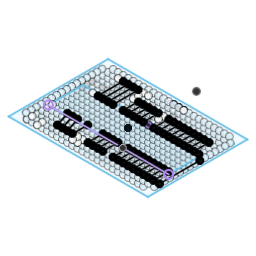
teensy_circuit_board v7 (Autodesk Fusion 360 design; units mm, degrees)
Autodesk Fusion 360 part; units mm, degrees
sketch "board" plane through (0, 0, 0) normal (0, 0, 1) x (1, 0, 0)
  circle A0 centre (-29.2, -21.5) radius 0.5
  line L0 (-35, 25) -> (35, 25)
  line L1 (35, 25) -> (35, -25)
  line L2 (35, -25) -> (-35, -25)
  line L3 (-35, -25) -> (-35, 25)
  circle A1 centre (-26.66, -21.5) radius 0.5
  circle A2 centre (-24.12, -21.5) radius 0.5
  circle A3 centre (-21.58, -21.5) radius 0.5
  circle A4 centre (-19.04, -21.5) radius 0.5
  circle A5 centre (-16.5, -21.5) radius 0.5
  circle A6 centre (-13.96, -21.5) radius 0.5
  circle A7 centre (-11.42, -21.5) radius 0.5
  circle A8 centre (-8.88, -21.5) radius 0.5
  circle A9 centre (-6.34, -21.5) radius 0.5
  circle A10 centre (-3.8, -21.5) radius 0.5
  circle A11 centre (-1.26, -21.5) radius 0.5
  circle A12 centre (1.28, -21.5) radius 0.5
  circle A13 centre (3.82, -21.5) radius 0.5
  circle A14 centre (6.36, -21.5) radius 0.5
  circle A15 centre (8.9, -21.5) radius 0.5
  circle A16 centre (11.44, -21.5) radius 0.5
  circle A17 centre (13.98, -21.5) radius 0.5
  circle A18 centre (16.52, -21.5) radius 0.5
  circle A19 centre (19.06, -21.5) radius 0.5
  circle A20 centre (21.6, -21.5) radius 0.5
  circle A21 centre (24.14, -21.5) radius 0.5
  circle A22 centre (26.68, -21.5) radius 0.5
  circle A23 centre (29.22, -21.5) radius 0.5
  circle A24 centre (-29.2, -18.96) radius 0.5
  circle A25 centre (-26.66, -18.96) radius 0.5
  circle A26 centre (-24.12, -18.96) radius 0.5
  circle A27 centre (-21.58, -18.96) radius 0.5
  circle A28 centre (-19.04, -18.96) radius 0.5
  circle A29 centre (-16.5, -18.96) radius 0.5
  circle A30 centre (-13.96, -18.96) radius 0.5
  circle A31 centre (-11.42, -18.96) radius 0.5
  circle A32 centre (-8.88, -18.96) radius 0.5
  circle A33 centre (-6.34, -18.96) radius 0.5
  circle A34 centre (-3.8, -18.96) radius 0.5
  circle A35 centre (-1.26, -18.96) radius 0.5
  circle A36 centre (1.28, -18.96) radius 0.5
  circle A37 centre (3.82, -18.96) radius 0.5
  circle A38 centre (6.36, -18.96) radius 0.5
  circle A39 centre (8.9, -18.96) radius 0.5
  circle A40 centre (11.44, -18.96) radius 0.5
  circle A41 centre (13.98, -18.96) radius 0.5
  circle A42 centre (16.52, -18.96) radius 0.5
  circle A43 centre (19.06, -18.96) radius 0.5
  circle A44 centre (21.6, -18.96) radius 0.5
  circle A45 centre (24.14, -18.96) radius 0.5
  circle A46 centre (26.68, -18.96) radius 0.5
  circle A47 centre (29.22, -18.96) radius 0.5
  circle A48 centre (-29.2, -16.42) radius 0.5
  circle A49 centre (-26.66, -16.42) radius 0.5
  circle A50 centre (-24.12, -16.42) radius 0.5
  circle A51 centre (-21.58, -16.42) radius 0.5
  circle A52 centre (-19.04, -16.42) radius 0.5
  circle A53 centre (-16.5, -16.42) radius 0.5
  circle A54 centre (-13.96, -16.42) radius 0.5
  circle A55 centre (-11.42, -16.42) radius 0.5
  circle A56 centre (-8.88, -16.42) radius 0.5
  circle A57 centre (-6.34, -16.42) radius 0.5
  circle A58 centre (-3.8, -16.42) radius 0.5
  circle A59 centre (-1.26, -16.42) radius 0.5
  circle A60 centre (1.28, -16.42) radius 0.5
  circle A61 centre (3.82, -16.42) radius 0.5
  circle A62 centre (6.36, -16.42) radius 0.5
  circle A63 centre (8.9, -16.42) radius 0.5
  circle A64 centre (11.44, -16.42) radius 0.5
  circle A65 centre (13.98, -16.42) radius 0.5
  circle A66 centre (16.52, -16.42) radius 0.5
  circle A67 centre (19.06, -16.42) radius 0.5
  circle A68 centre (21.6, -16.42) radius 0.5
  circle A69 centre (24.14, -16.42) radius 0.5
  circle A70 centre (26.68, -16.42) radius 0.5
  circle A71 centre (29.22, -16.42) radius 0.5
  circle A72 centre (-29.2, -13.88) radius 0.5
  circle A73 centre (-26.66, -13.88) radius 0.5
  circle A74 centre (-24.12, -13.88) radius 0.5
  circle A75 centre (-21.58, -13.88) radius 0.5
  circle A76 centre (-19.04, -13.88) radius 0.5
  circle A77 centre (-16.5, -13.88) radius 0.5
  circle A78 centre (-13.96, -13.88) radius 0.5
  circle A79 centre (-11.42, -13.88) radius 0.5
  circle A80 centre (-8.88, -13.88) radius 0.5
  circle A81 centre (-6.34, -13.88) radius 0.5
  circle A82 centre (-3.8, -13.88) radius 0.5
  circle A83 centre (-1.26, -13.88) radius 0.5
  circle A84 centre (1.28, -13.88) radius 0.5
  circle A85 centre (3.82, -13.88) radius 0.5
  circle A86 centre (6.36, -13.88) radius 0.5
  circle A87 centre (8.9, -13.88) radius 0.5
  circle A88 centre (11.44, -13.88) radius 0.5
  circle A89 centre (13.98, -13.88) radius 0.5
  circle A90 centre (16.52, -13.88) radius 0.5
  circle A91 centre (19.06, -13.88) radius 0.5
  circle A92 centre (21.6, -13.88) radius 0.5
  circle A93 centre (24.14, -13.88) radius 0.5
  circle A94 centre (26.68, -13.88) radius 0.5
  circle A95 centre (29.22, -13.88) radius 0.5
  circle A96 centre (-29.2, -11.34) radius 0.5
  circle A97 centre (-26.66, -11.34) radius 0.5
  circle A98 centre (-24.12, -11.34) radius 0.5
  circle A99 centre (-21.58, -11.34) radius 0.5
  circle A100 centre (-19.04, -11.34) radius 0.5
  circle A101 centre (-16.5, -11.34) radius 0.5
  circle A102 centre (-13.96, -11.34) radius 0.5
  circle A103 centre (-11.42, -11.34) radius 0.5
  circle A104 centre (-8.88, -11.34) radius 0.5
  circle A105 centre (-6.34, -11.34) radius 0.5
  circle A106 centre (-3.8, -11.34) radius 0.5
  circle A107 centre (-1.26, -11.34) radius 0.5
  circle A108 centre (1.28, -11.34) radius 0.5
  circle A109 centre (3.82, -11.34) radius 0.5
  circle A110 centre (6.36, -11.34) radius 0.5
  circle A111 centre (8.9, -11.34) radius 0.5
  circle A112 centre (11.44, -11.34) radius 0.5
  circle A113 centre (13.98, -11.34) radius 0.5
  circle A114 centre (16.52, -11.34) radius 0.5
  circle A115 centre (19.06, -11.34) radius 0.5
  circle A116 centre (21.6, -11.34) radius 0.5
  circle A117 centre (24.14, -11.34) radius 0.5
  circle A118 centre (26.68, -11.34) radius 0.5
  circle A119 centre (29.22, -11.34) radius 0.5
  circle A120 centre (-29.2, -8.8) radius 0.5
  circle A121 centre (-26.66, -8.8) radius 0.5
  circle A122 centre (-24.12, -8.8) radius 0.5
  circle A123 centre (-21.58, -8.8) radius 0.5
  circle A124 centre (-19.04, -8.8) radius 0.5
  circle A125 centre (-16.5, -8.8) radius 0.5
  circle A126 centre (-13.96, -8.8) radius 0.5
  circle A127 centre (-11.42, -8.8) radius 0.5
  circle A128 centre (-8.88, -8.8) radius 0.5
  circle A129 centre (-6.34, -8.8) radius 0.5
  circle A130 centre (-3.8, -8.8) radius 0.5
  circle A131 centre (-1.26, -8.8) radius 0.5
  circle A132 centre (1.28, -8.8) radius 0.5
  circle A133 centre (3.82, -8.8) radius 0.5
  circle A134 centre (6.36, -8.8) radius 0.5
  circle A135 centre (8.9, -8.8) radius 0.5
  circle A136 centre (11.44, -8.8) radius 0.5
  circle A137 centre (13.98, -8.8) radius 0.5
  circle A138 centre (16.52, -8.8) radius 0.5
  circle A139 centre (19.06, -8.8) radius 0.5
  circle A140 centre (21.6, -8.8) radius 0.5
  circle A141 centre (24.14, -8.8) radius 0.5
  circle A142 centre (26.68, -8.8) radius 0.5
  circle A143 centre (29.22, -8.8) radius 0.5
  circle A144 centre (-29.2, -6.26) radius 0.5
  circle A145 centre (-26.66, -6.26) radius 0.5
  circle A146 centre (-24.12, -6.26) radius 0.5
  circle A147 centre (-21.58, -6.26) radius 0.5
  circle A148 centre (-19.04, -6.26) radius 0.5
  circle A149 centre (-16.5, -6.26) radius 0.5
  circle A150 centre (-13.96, -6.26) radius 0.5
  circle A151 centre (-11.42, -6.26) radius 0.5
  circle A152 centre (-8.88, -6.26) radius 0.5
  circle A153 centre (-6.34, -6.26) radius 0.5
  circle A154 centre (-3.8, -6.26) radius 0.5
  circle A155 centre (-1.26, -6.26) radius 0.5
  circle A156 centre (1.28, -6.26) radius 0.5
  circle A157 centre (3.82, -6.26) radius 0.5
  circle A158 centre (6.36, -6.26) radius 0.5
  circle A159 centre (8.9, -6.26) radius 0.5
  circle A160 centre (11.44, -6.26) radius 0.5
  circle A161 centre (13.98, -6.26) radius 0.5
  circle A162 centre (16.52, -6.26) radius 0.5
  circle A163 centre (19.06, -6.26) radius 0.5
  circle A164 centre (21.6, -6.26) radius 0.5
  circle A165 centre (24.14, -6.26) radius 0.5
  circle A166 centre (26.68, -6.26) radius 0.5
  circle A167 centre (29.22, -6.26) radius 0.5
  circle A168 centre (-29.2, -3.72) radius 0.5
  circle A169 centre (-26.66, -3.72) radius 0.5
  circle A170 centre (-24.12, -3.72) radius 0.5
  circle A171 centre (-21.58, -3.72) radius 0.5
  circle A172 centre (-19.04, -3.72) radius 0.5
  circle A173 centre (-16.5, -3.72) radius 0.5
  circle A174 centre (-13.96, -3.72) radius 0.5
  circle A175 centre (-11.42, -3.72) radius 0.5
  circle A176 centre (-8.88, -3.72) radius 0.5
  circle A177 centre (-6.34, -3.72) radius 0.5
  circle A178 centre (-3.8, -3.72) radius 0.5
  circle A179 centre (-1.26, -3.72) radius 0.5
  circle A180 centre (1.28, -3.72) radius 0.5
  circle A181 centre (3.82, -3.72) radius 0.5
  circle A182 centre (6.36, -3.72) radius 0.5
  circle A183 centre (8.9, -3.72) radius 0.5
  circle A184 centre (11.44, -3.72) radius 0.5
  circle A185 centre (13.98, -3.72) radius 0.5
  circle A186 centre (16.52, -3.72) radius 0.5
  circle A187 centre (19.06, -3.72) radius 0.5
  circle A188 centre (21.6, -3.72) radius 0.5
  circle A189 centre (24.14, -3.72) radius 0.5
  circle A190 centre (26.68, -3.72) radius 0.5
  circle A191 centre (29.22, -3.72) radius 0.5
  circle A192 centre (-29.2, -1.18) radius 0.5
  circle A193 centre (-26.66, -1.18) radius 0.5
  circle A194 centre (-24.12, -1.18) radius 0.5
  circle A195 centre (-21.58, -1.18) radius 0.5
  circle A196 centre (-19.04, -1.18) radius 0.5
  circle A197 centre (-16.5, -1.18) radius 0.5
  circle A198 centre (-13.96, -1.18) radius 0.5
  circle A199 centre (-11.42, -1.18) radius 0.5
  circle A200 centre (-8.88, -1.18) radius 0.5
  circle A201 centre (-6.34, -1.18) radius 0.5
  circle A202 centre (-3.8, -1.18) radius 0.5
  circle A203 centre (-1.26, -1.18) radius 0.5
  circle A204 centre (1.28, -1.18) radius 0.5
  circle A205 centre (3.82, -1.18) radius 0.5
  circle A206 centre (6.36, -1.18) radius 0.5
  circle A207 centre (8.9, -1.18) radius 0.5
  circle A208 centre (11.44, -1.18) radius 0.5
  circle A209 centre (13.98, -1.18) radius 0.5
  circle A210 centre (16.52, -1.18) radius 0.5
  circle A211 centre (19.06, -1.18) radius 0.5
  circle A212 centre (21.6, -1.18) radius 0.5
  circle A213 centre (24.14, -1.18) radius 0.5
  circle A214 centre (26.68, -1.18) radius 0.5
  circle A215 centre (29.22, -1.18) radius 0.5
  circle A216 centre (-29.2, 1.36) radius 0.5
  circle A217 centre (-26.66, 1.36) radius 0.5
  circle A218 centre (-24.12, 1.36) radius 0.5
  circle A219 centre (-21.58, 1.36) radius 0.5
  circle A220 centre (-19.04, 1.36) radius 0.5
  circle A221 centre (-16.5, 1.36) radius 0.5
  circle A222 centre (-13.96, 1.36) radius 0.5
  circle A223 centre (-11.42, 1.36) radius 0.5
  circle A224 centre (-8.88, 1.36) radius 0.5
  circle A225 centre (-6.34, 1.36) radius 0.5
  circle A226 centre (-3.8, 1.36) radius 0.5
  circle A227 centre (-1.26, 1.36) radius 0.5
  circle A228 centre (1.28, 1.36) radius 0.5
  circle A229 centre (3.82, 1.36) radius 0.5
  circle A230 centre (6.36, 1.36) radius 0.5
  circle A231 centre (8.9, 1.36) radius 0.5
  circle A232 centre (11.44, 1.36) radius 0.5
  circle A233 centre (13.98, 1.36) radius 0.5
  circle A234 centre (16.52, 1.36) radius 0.5
  circle A235 centre (19.06, 1.36) radius 0.5
  circle A236 centre (21.6, 1.36) radius 0.5
  circle A237 centre (24.14, 1.36) radius 0.5
  circle A238 centre (26.68, 1.36) radius 0.5
  circle A239 centre (29.22, 1.36) radius 0.5
  circle A240 centre (-29.2, 3.9) radius 0.5
  circle A241 centre (-26.66, 3.9) radius 0.5
  circle A242 centre (-24.12, 3.9) radius 0.5
  circle A243 centre (-21.58, 3.9) radius 0.5
  circle A244 centre (-19.04, 3.9) radius 0.5
  circle A245 centre (-16.5, 3.9) radius 0.5
  circle A246 centre (-13.96, 3.9) radius 0.5
  circle A247 centre (-11.42, 3.9) radius 0.5
  circle A248 centre (-8.88, 3.9) radius 0.5
  circle A249 centre (-6.34, 3.9) radius 0.5
  circle A250 centre (-3.8, 3.9) radius 0.5
  circle A251 centre (-1.26, 3.9) radius 0.5
  circle A252 centre (1.28, 3.9) radius 0.5
  circle A253 centre (3.82, 3.9) radius 0.5
  circle A254 centre (6.36, 3.9) radius 0.5
  circle A255 centre (8.9, 3.9) radius 0.5
  circle A256 centre (11.44, 3.9) radius 0.5
  circle A257 centre (13.98, 3.9) radius 0.5
  circle A258 centre (16.52, 3.9) radius 0.5
  circle A259 centre (19.06, 3.9) radius 0.5
  circle A260 centre (21.6, 3.9) radius 0.5
  circle A261 centre (24.14, 3.9) radius 0.5
  circle A262 centre (26.68, 3.9) radius 0.5
  circle A263 centre (29.22, 3.9) radius 0.5
  circle A264 centre (-29.2, 6.44) radius 0.5
  circle A265 centre (-26.66, 6.44) radius 0.5
  circle A266 centre (-24.12, 6.44) radius 0.5
  circle A267 centre (-21.58, 6.44) radius 0.5
  circle A268 centre (-19.04, 6.44) radius 0.5
  circle A269 centre (-16.5, 6.44) radius 0.5
  circle A270 centre (-13.96, 6.44) radius 0.5
  circle A271 centre (-11.42, 6.44) radius 0.5
  circle A272 centre (-8.88, 6.44) radius 0.5
  circle A273 centre (-6.34, 6.44) radius 0.5
  circle A274 centre (-3.8, 6.44) radius 0.5
  circle A275 centre (-1.26, 6.44) radius 0.5
  circle A276 centre (1.28, 6.44) radius 0.5
  circle A277 centre (3.82, 6.44) radius 0.5
  circle A278 centre (6.36, 6.44) radius 0.5
  circle A279 centre (8.9, 6.44) radius 0.5
  circle A280 centre (11.44, 6.44) radius 0.5
  circle A281 centre (13.98, 6.44) radius 0.5
  circle A282 centre (16.52, 6.44) radius 0.5
  circle A283 centre (19.06, 6.44) radius 0.5
  circle A284 centre (21.6, 6.44) radius 0.5
  circle A285 centre (24.14, 6.44) radius 0.5
  circle A286 centre (26.68, 6.44) radius 0.5
  circle A287 centre (29.22, 6.44) radius 0.5
  circle A288 centre (-29.2, 8.98) radius 0.5
  circle A289 centre (-26.66, 8.98) radius 0.5
  circle A290 centre (-24.12, 8.98) radius 0.5
  circle A291 centre (-21.58, 8.98) radius 0.5
  circle A292 centre (-19.04, 8.98) radius 0.5
  circle A293 centre (-16.5, 8.98) radius 0.5
  circle A294 centre (-13.96, 8.98) radius 0.5
  circle A295 centre (-11.42, 8.98) radius 0.5
  circle A296 centre (-8.88, 8.98) radius 0.5
  circle A297 centre (-6.34, 8.98) radius 0.5
  circle A298 centre (-3.8, 8.98) radius 0.5
  circle A299 centre (-1.26, 8.98) radius 0.5
  circle A300 centre (1.28, 8.98) radius 0.5
  circle A301 centre (3.82, 8.98) radius 0.5
  circle A302 centre (6.36, 8.98) radius 0.5
  circle A303 centre (8.9, 8.98) radius 0.5
  circle A304 centre (11.44, 8.98) radius 0.5
  circle A305 centre (13.98, 8.98) radius 0.5
  circle A306 centre (16.52, 8.98) radius 0.5
  circle A307 centre (19.06, 8.98) radius 0.5
  circle A308 centre (21.6, 8.98) radius 0.5
  circle A309 centre (24.14, 8.98) radius 0.5
  circle A310 centre (26.68, 8.98) radius 0.5
  circle A311 centre (29.22, 8.98) radius 0.5
  circle A312 centre (-29.2, 11.52) radius 0.5
  circle A313 centre (-26.66, 11.52) radius 0.5
  circle A314 centre (-24.12, 11.52) radius 0.5
  circle A315 centre (-21.58, 11.52) radius 0.5
  circle A316 centre (-19.04, 11.52) radius 0.5
  circle A317 centre (-16.5, 11.52) radius 0.5
  circle A318 centre (-13.96, 11.52) radius 0.5
  circle A319 centre (-11.42, 11.52) radius 0.5
  circle A320 centre (-8.88, 11.52) radius 0.5
  circle A321 centre (-6.34, 11.52) radius 0.5
  circle A322 centre (-3.8, 11.52) radius 0.5
  circle A323 centre (-1.26, 11.52) radius 0.5
  circle A324 centre (1.28, 11.52) radius 0.5
  circle A325 centre (3.82, 11.52) radius 0.5
  circle A326 centre (6.36, 11.52) radius 0.5
  circle A327 centre (8.9, 11.52) radius 0.5
  circle A328 centre (11.44, 11.52) radius 0.5
  circle A329 centre (13.98, 11.52) radius 0.5
  circle A330 centre (16.52, 11.52) radius 0.5
  circle A331 centre (19.06, 11.52) radius 0.5
  circle A332 centre (21.6, 11.52) radius 0.5
  circle A333 centre (24.14, 11.52) radius 0.5
  circle A334 centre (26.68, 11.52) radius 0.5
  circle A335 centre (29.22, 11.52) radius 0.5
  circle A336 centre (-29.2, 14.06) radius 0.5
  circle A337 centre (-26.66, 14.06) radius 0.5
  circle A338 centre (-24.12, 14.06) radius 0.5
  circle A339 centre (-21.58, 14.06) radius 0.5
  circle A340 centre (-19.04, 14.06) radius 0.5
  circle A341 centre (-16.5, 14.06) radius 0.5
  circle A342 centre (-13.96, 14.06) radius 0.5
  circle A343 centre (-11.42, 14.06) radius 0.5
  circle A344 centre (-8.88, 14.06) radius 0.5
  circle A345 centre (-6.34, 14.06) radius 0.5
  circle A346 centre (-3.8, 14.06) radius 0.5
  circle A347 centre (-1.26, 14.06) radius 0.5
  circle A348 centre (1.28, 14.06) radius 0.5
  circle A349 centre (3.82, 14.06) radius 0.5
  circle A350 centre (6.36, 14.06) radius 0.5
  circle A351 centre (8.9, 14.06) radius 0.5
  circle A352 centre (11.44, 14.06) radius 0.5
  circle A353 centre (13.98, 14.06) radius 0.5
  circle A354 centre (16.52, 14.06) radius 0.5
  circle A355 centre (19.06, 14.06) radius 0.5
  circle A356 centre (21.6, 14.06) radius 0.5
  circle A357 centre (24.14, 14.06) radius 0.5
  circle A358 centre (26.68, 14.06) radius 0.5
  circle A359 centre (29.22, 14.06) radius 0.5
  circle A360 centre (-29.2, 16.6) radius 0.5
  circle A361 centre (-26.66, 16.6) radius 0.5
  circle A362 centre (-24.12, 16.6) radius 0.5
  circle A363 centre (-21.58, 16.6) radius 0.5
  circle A364 centre (-19.04, 16.6) radius 0.5
  circle A365 centre (-16.5, 16.6) radius 0.5
  circle A366 centre (-13.96, 16.6) radius 0.5
  circle A367 centre (-11.42, 16.6) radius 0.5
  circle A368 centre (-8.88, 16.6) radius 0.5
  circle A369 centre (-6.34, 16.6) radius 0.5
  circle A370 centre (-3.8, 16.6) radius 0.5
  circle A371 centre (-1.26, 16.6) radius 0.5
  circle A372 centre (1.28, 16.6) radius 0.5
  circle A373 centre (3.82, 16.6) radius 0.5
  circle A374 centre (6.36, 16.6) radius 0.5
  circle A375 centre (8.9, 16.6) radius 0.5
  circle A376 centre (11.44, 16.6) radius 0.5
  circle A377 centre (13.98, 16.6) radius 0.5
  circle A378 centre (16.52, 16.6) radius 0.5
  circle A379 centre (19.06, 16.6) radius 0.5
  circle A380 centre (21.6, 16.6) radius 0.5
  circle A381 centre (24.14, 16.6) radius 0.5
  circle A382 centre (26.68, 16.6) radius 0.5
  circle A383 centre (29.22, 16.6) radius 0.5
  circle A384 centre (-29.2, 19.14) radius 0.5
  circle A385 centre (-26.66, 19.14) radius 0.5
  circle A386 centre (-24.12, 19.14) radius 0.5
  circle A387 centre (-21.58, 19.14) radius 0.5
  circle A388 centre (-19.04, 19.14) radius 0.5
  circle A389 centre (-16.5, 19.14) radius 0.5
  circle A390 centre (-13.96, 19.14) radius 0.5
  circle A391 centre (-11.42, 19.14) radius 0.5
  circle A392 centre (-8.88, 19.14) radius 0.5
  circle A393 centre (-6.34, 19.14) radius 0.5
  circle A394 centre (-3.8, 19.14) radius 0.5
  circle A395 centre (-1.26, 19.14) radius 0.5
  circle A396 centre (1.28, 19.14) radius 0.5
  circle A397 centre (3.82, 19.14) radius 0.5
  circle A398 centre (6.36, 19.14) radius 0.5
  circle A399 centre (8.9, 19.14) radius 0.5
  circle A400 centre (11.44, 19.14) radius 0.5
  circle A401 centre (13.98, 19.14) radius 0.5
  circle A402 centre (16.52, 19.14) radius 0.5
  circle A403 centre (19.06, 19.14) radius 0.5
  circle A404 centre (21.6, 19.14) radius 0.5
  circle A405 centre (24.14, 19.14) radius 0.5
  circle A406 centre (26.68, 19.14) radius 0.5
  circle A407 centre (29.22, 19.14) radius 0.5
  circle A408 centre (-29.2, 21.68) radius 0.5
  circle A409 centre (-26.66, 21.68) radius 0.5
  circle A410 centre (-24.12, 21.68) radius 0.5
  circle A411 centre (-21.58, 21.68) radius 0.5
  circle A412 centre (-19.04, 21.68) radius 0.5
  circle A413 centre (-16.5, 21.68) radius 0.5
  circle A414 centre (-13.96, 21.68) radius 0.5
  circle A415 centre (-11.42, 21.68) radius 0.5
  circle A416 centre (-8.88, 21.68) radius 0.5
  circle A417 centre (-6.34, 21.68) radius 0.5
  circle A418 centre (-3.8, 21.68) radius 0.5
  circle A419 centre (-1.26, 21.68) radius 0.5
  circle A420 centre (1.28, 21.68) radius 0.5
  circle A421 centre (3.82, 21.68) radius 0.5
  circle A422 centre (6.36, 21.68) radius 0.5
  circle A423 centre (8.9, 21.68) radius 0.5
  circle A424 centre (11.44, 21.68) radius 0.5
  circle A425 centre (13.98, 21.68) radius 0.5
  circle A426 centre (16.52, 21.68) radius 0.5
  circle A427 centre (19.06, 21.68) radius 0.5
  circle A428 centre (21.6, 21.68) radius 0.5
  circle A429 centre (24.14, 21.68) radius 0.5
  circle A430 centre (26.68, 21.68) radius 0.5
  circle A431 centre (29.22, 21.68) radius 0.5
  line L4 (-33.3, 18.5) -> (-33.3, 19.8)
  line L5 (-33.3, 19.8) -> (-32.2, 19.8)
  line L6 (-33.3, 18.5) -> (-32.2, 18.5)
  arc A432 (-32.2, 18.5) -> (-32.2, 19.8) centre (-32.2, 19.15) ccw
  arc A433 (-32.2, 15.96) -> (-32.2, 17.26) centre (-32.2, 16.61) ccw
  line L7 (-33.3, 15.96) -> (-32.2, 15.96)
  line L8 (-33.3, 15.96) -> (-33.3, 17.26)
  line L9 (-33.3, 17.26) -> (-32.2, 17.26)
  arc A434 (-32.2, 13.42) -> (-32.2, 14.72) centre (-32.2, 14.07) ccw
  line L10 (-33.3, 13.42) -> (-32.2, 13.42)
  line L11 (-33.3, 13.42) -> (-33.3, 14.72)
  line L12 (-33.3, 14.72) -> (-32.2, 14.72)
  arc A435 (-32.2, 10.88) -> (-32.2, 12.18) centre (-32.2, 11.53) ccw
  line L13 (-33.3, 10.88) -> (-32.2, 10.88)
  line L14 (-33.3, 10.88) -> (-33.3, 12.18)
  line L15 (-33.3, 12.18) -> (-32.2, 12.18)
  arc A436 (-32.2, 8.34) -> (-32.2, 9.64) centre (-32.2, 8.99) ccw
  line L16 (-33.3, 8.34) -> (-32.2, 8.34)
  line L17 (-33.3, 8.34) -> (-33.3, 9.64)
  line L18 (-33.3, 9.64) -> (-32.2, 9.64)
  arc A437 (-32.2, 5.8) -> (-32.2, 7.1) centre (-32.2, 6.45) ccw
  line L19 (-33.3, 5.8) -> (-32.2, 5.8)
  line L20 (-33.3, 5.8) -> (-33.3, 7.1)
  line L21 (-33.3, 7.1) -> (-32.2, 7.1)
  arc A438 (-32.2, 3.26) -> (-32.2, 4.56) centre (-32.2, 3.91) ccw
  line L22 (-33.3, 3.26) -> (-32.2, 3.26)
  line L23 (-33.3, 3.26) -> (-33.3, 4.56)
  line L24 (-33.3, 4.56) -> (-32.2, 4.56)
  arc A439 (-32.2, 0.72) -> (-32.2, 2.02) centre (-32.2, 1.37) ccw
  line L25 (-33.3, 0.72) -> (-32.2, 0.72)
  line L26 (-33.3, 0.72) -> (-33.3, 2.02)
  line L27 (-33.3, 2.02) -> (-32.2, 2.02)
  arc A440 (-32.2, -1.82) -> (-32.2, -0.52) centre (-32.2, -1.17) ccw
  line L28 (-33.3, -1.82) -> (-32.2, -1.82)
  line L29 (-33.3, -1.82) -> (-33.3, -0.52)
  line L30 (-33.3, -0.52) -> (-32.2, -0.52)
  arc A441 (-32.2, -4.36) -> (-32.2, -3.06) centre (-32.2, -3.71) ccw
  line L31 (-33.3, -4.36) -> (-32.2, -4.36)
  line L32 (-33.3, -4.36) -> (-33.3, -3.06)
  line L33 (-33.3, -3.06) -> (-32.2, -3.06)
  arc A442 (-32.2, -6.9) -> (-32.2, -5.6) centre (-32.2, -6.25) ccw
  line L34 (-33.3, -6.9) -> (-32.2, -6.9)
  line L35 (-33.3, -6.9) -> (-33.3, -5.6)
  line L36 (-33.3, -5.6) -> (-32.2, -5.6)
  arc A443 (-32.2, -9.44) -> (-32.2, -8.14) centre (-32.2, -8.79) ccw
  line L37 (-33.3, -9.44) -> (-32.2, -9.44)
  line L38 (-33.3, -9.44) -> (-33.3, -8.14)
  line L39 (-33.3, -8.14) -> (-32.2, -8.14)
  arc A444 (-32.2, -11.98) -> (-32.2, -10.68) centre (-32.2, -11.33) ccw
  line L40 (-33.3, -11.98) -> (-32.2, -11.98)
  line L41 (-33.3, -11.98) -> (-33.3, -10.68)
  line L42 (-33.3, -10.68) -> (-32.2, -10.68)
  arc A445 (-32.2, -14.52) -> (-32.2, -13.22) centre (-32.2, -13.87) ccw
  line L43 (-33.3, -14.52) -> (-32.2, -14.52)
  line L44 (-33.3, -14.52) -> (-33.3, -13.22)
  line L45 (-33.3, -13.22) -> (-32.2, -13.22)
  arc A446 (-32.2, -17.06) -> (-32.2, -15.76) centre (-32.2, -16.41) ccw
  line L46 (-33.3, -17.06) -> (-32.2, -17.06)
  line L47 (-33.3, -17.06) -> (-33.3, -15.76)
  line L48 (-33.3, -15.76) -> (-32.2, -15.76)
  arc A447 (-32.2, -19.6) -> (-32.2, -18.3) centre (-32.2, -18.95) ccw
  line L49 (-33.3, -19.6) -> (-32.2, -19.6)
  line L50 (-33.3, -19.6) -> (-33.3, -18.3)
  line L51 (-33.3, -18.3) -> (-32.2, -18.3)
  line L52 (33.3, -5.6) -> (32.2, -5.6)
  line L53 (33.3, 15.96) -> (32.2, 15.96)
  line L54 (33.3, 13.42) -> (32.2, 13.42)
  arc A448 (32.2, -13.22) -> (32.2, -14.52) centre (32.2, -13.87) ccw
  arc A449 (32.2, 19.8) -> (32.2, 18.5) centre (32.2, 19.15) ccw
  line L55 (33.3, -19.6) -> (33.3, -18.3)
  line L56 (33.3, 19.8) -> (32.2, 19.8)
  line L57 (33.3, 18.5) -> (32.2, 18.5)
  line L58 (33.3, 18.5) -> (33.3, 19.8)
  line L59 (33.3, 13.42) -> (33.3, 14.72)
  line L60 (33.3, -11.98) -> (33.3, -10.68)
  line L61 (33.3, -17.06) -> (32.2, -17.06)
  arc A450 (32.2, -10.68) -> (32.2, -11.98) centre (32.2, -11.33) ccw
  line L62 (33.3, 0.72) -> (33.3, 2.02)
  line L63 (33.3, 8.34) -> (33.3, 9.64)
  arc A451 (32.2, -8.14) -> (32.2, -9.44) centre (32.2, -8.79) ccw
  line L64 (33.3, -9.44) -> (33.3, -8.14)
  line L65 (33.3, -8.14) -> (32.2, -8.14)
  line L66 (33.3, 10.88) -> (32.2, 10.88)
  line L67 (33.3, -1.82) -> (32.2, -1.82)
  arc A452 (32.2, 2.02) -> (32.2, 0.72) centre (32.2, 1.37) ccw
  line L68 (33.3, -6.9) -> (32.2, -6.9)
  line L69 (33.3, -4.36) -> (32.2, -4.36)
  line L70 (33.3, 3.26) -> (33.3, 4.56)
  arc A453 (32.2, -5.6) -> (32.2, -6.9) centre (32.2, -6.25) ccw
  line L71 (33.3, 5.8) -> (33.3, 7.1)
  line L72 (33.3, -4.36) -> (33.3, -3.06)
  line L73 (33.3, 9.64) -> (32.2, 9.64)
  line L74 (33.3, 0.72) -> (32.2, 0.72)
  line L75 (33.3, 3.26) -> (32.2, 3.26)
  arc A454 (32.2, 9.64) -> (32.2, 8.34) centre (32.2, 8.99) ccw
  line L76 (33.3, -1.82) -> (33.3, -0.52)
  arc A455 (32.2, -0.52) -> (32.2, -1.82) centre (32.2, -1.17) ccw
  arc A456 (32.2, 4.56) -> (32.2, 3.26) centre (32.2, 3.91) ccw
  line L77 (33.3, 5.8) -> (32.2, 5.8)
  line L78 (33.3, -3.06) -> (32.2, -3.06)
  line L79 (33.3, -9.44) -> (32.2, -9.44)
  line L80 (33.3, 7.1) -> (32.2, 7.1)
  line L81 (33.3, 2.02) -> (32.2, 2.02)
  line L82 (33.3, -6.9) -> (33.3, -5.6)
  line L83 (33.3, -10.68) -> (32.2, -10.68)
  arc A457 (32.2, -3.06) -> (32.2, -4.36) centre (32.2, -3.71) ccw
  line L84 (33.3, 8.34) -> (32.2, 8.34)
  arc A458 (32.2, 7.1) -> (32.2, 5.8) centre (32.2, 6.45) ccw
  line L85 (33.3, -0.52) -> (32.2, -0.52)
  line L86 (33.3, 4.56) -> (32.2, 4.56)
  arc A459 (32.2, -15.76) -> (32.2, -17.06) centre (32.2, -16.41) ccw
  line L87 (33.3, -17.06) -> (33.3, -15.76)
  line L88 (33.3, -11.98) -> (32.2, -11.98)
  line L89 (33.3, 15.96) -> (33.3, 17.26)
  line L90 (33.3, -14.52) -> (33.3, -13.22)
  line L91 (33.3, -19.6) -> (32.2, -19.6)
  line L92 (33.3, 10.88) -> (33.3, 12.18)
  line L93 (33.3, 17.26) -> (32.2, 17.26)
  arc A460 (32.2, 17.26) -> (32.2, 15.96) centre (32.2, 16.61) ccw
  line L94 (33.3, -14.52) -> (32.2, -14.52)
  line L95 (33.3, -15.76) -> (32.2, -15.76)
  arc A461 (32.2, -18.3) -> (32.2, -19.6) centre (32.2, -18.95) ccw
  line L96 (33.3, 12.18) -> (32.2, 12.18)
  line L97 (33.3, -13.22) -> (32.2, -13.22)
  line L98 (33.3, 14.72) -> (32.2, 14.72)
  arc A462 (32.2, 12.18) -> (32.2, 10.88) centre (32.2, 11.53) ccw
  arc A463 (32.2, 14.72) -> (32.2, 13.42) centre (32.2, 14.07) ccw
  line L99 (33.3, -18.3) -> (32.2, -18.3)
  dimension "d1" = 70
  dimension "d2" = 50
  constraint horizontal L0
  constraint perpendicular L0 L1
  constraint parallel L0 L2
  constraint parallel L1 L3
  measures "d1" distance of L1.end L2.end
  measures "d2" distance of L0.end L1.end
sketch "teensy" plane through (0, 0, 0) normal (0, 0, 1) x (1, 0, 0)
  line L0 (-30, 7.5) -> (30.389, 7.5)
  line L1 (30.389, 7.5) -> (30.389, -10)
  line L2 (30.389, -10) -> (-30, -10)
  line L3 (-30, -10) -> (-30, 7.5)
  dimension "d11" = 17.5
  constraint horizontal L0
  constraint vertical L1
  constraint horizontal L2
  constraint vertical L3
  measures "d11" distance of L0.start L2.end
extrude "Extrude1" add sketch "teensy" against normal blind 1
sketch "connectors" plane through (0, 0, 0) normal (0, 0, 1) x (1, 0, 0)
  line L0 (-30.5809, -18.0287) -> (-23.3364, -18.0287)
  line L1 (-23.3364, -18.0287) -> (-23.3364, -19.8573)
  line L2 (-23.3364, -19.8573) -> (-30.5809, -19.8573)
  line L3 (-30.5809, -19.8573) -> (-30.5809, -18.0287)
  line L4 (7.8469, -15.668) -> (20.3638, -15.668)
  line L5 (20.3638, -15.668) -> (20.3638, -17.3421)
  line L6 (20.3638, -17.3421) -> (7.8469, -17.3421)
  line L7 (7.8469, -17.3421) -> (7.8469, -15.668)
  line L8 (20.3638, -15.668) -> (32.4641, -15.668)
  line L9 (32.4641, -15.668) -> (32.4641, -17.3421)
  line L10 (32.4641, -17.3421) -> (20.3638, -17.3421)
  line L11 (20.3638, -17.3421) -> (20.3638, -15.668)
  line L12 (-12.5361, 15) -> (7.3504, 15)
  line L13 (7.3504, 15) -> (7.3504, 13.1148)
  line L14 (7.3504, 13.1148) -> (-12.5361, 13.1148)
  line L15 (-12.5361, 13.1148) -> (-12.5361, 15)
  line L16 (-25.3054, 20.2) -> (-10.5, 20.2)
  line L17 (-10.5, 20.2) -> (-10.5, 18.2)
  line L18 (-10.5, 18.2) -> (-25.3054, 18.2)
  line L19 (-25.3054, 18.2) -> (-25.3054, 20.2)
  line L20 (27.6639, 15) -> (8, 15)
  line L21 (8, 15) -> (8, 13)
  line L22 (8, 13) -> (27.6639, 13)
  line L23 (27.6639, 13) -> (27.6639, 15)
  line L24 (7.3729, -10) -> (5.2914, -10)
  line L25 (5.2914, -10) -> (5.2914, -7.7315)
  line L26 (5.2914, -7.7315) -> (7.3729, -7.7315)
  line L27 (7.3729, -7.7315) -> (7.3729, -10)
  line L28 (30.389, -10) -> (-30, -10)
  line L29 (7.5, 5.5) -> (5.3795, 5.5)
  line L30 (5.3795, 5.5) -> (5.3795, 7.3487)
  line L31 (5.3795, 7.3487) -> (7.5, 7.3487)
  line L32 (7.5, 7.3487) -> (7.5, 5.5)
  line L33 (0.407, 22.584) -> (7.354, 22.584)
  line L34 (7.354, 22.584) -> (7.354, 20.7177)
  line L35 (7.354, 20.7177) -> (0.407, 20.7177)
  line L36 (0.407, 20.7177) -> (0.407, 22.584)
  line L37 (-20.1625, -15.471) -> (5.1467, -15.471)
  line L38 (5.1467, -15.471) -> (5.1467, -17.5368)
  line L39 (5.1467, -17.5368) -> (-20.1625, -17.5368)
  line L40 (-20.1625, -17.5368) -> (-20.1625, -15.471)
  constraint horizontal L0
  constraint vertical L1
  constraint horizontal L2
  constraint vertical L3
  constraint horizontal L4
  constraint vertical L5
  constraint horizontal L6
  constraint vertical L7
  constraint horizontal L8
  constraint vertical L9
  constraint horizontal L10
  constraint vertical L11
  constraint horizontal L12
  constraint vertical L13
  constraint horizontal L14
  constraint vertical L15
  constraint horizontal L16
  constraint vertical L17
  constraint horizontal L18
  constraint vertical L19
  constraint horizontal L20
  constraint vertical L21
  constraint horizontal L22
  constraint vertical L23
  constraint horizontal L24
  constraint vertical L25
  constraint horizontal L26
  constraint vertical L27
  constraint coincident L24.start L28
  constraint horizontal L29
  constraint vertical L30
  constraint horizontal L31
  constraint vertical L32
  constraint horizontal L33
  constraint vertical L34
  constraint horizontal L35
  constraint vertical L36
  constraint horizontal L37
  constraint vertical L38
  constraint horizontal L39
  constraint vertical L40
sketch "direct_solder" plane through (0, 0, 0) normal (0, 0, 1) x (1, 0, 0)
  line L0 (29.22, 6.44) -> (32.2, 3.91)
  line L1 (-21.58, 19.14) -> (-21.58, 6.44)
  line L2 (-19.04, 19.14) -> (-19.04, 6.44)
  line L3 (-16.5, 19.14) -> (-16.5, 6.44)
  line L4 (-13.96, 19.14) -> (-13.96, 6.44)
  line L5 (6.36, 14.06) -> (6.36, 6.44)
  line L6 (8.9, 14.06) -> (8.9, 6.44)
  line L7 (11.44, 14.06) -> (11.44, 6.44)
  line L8 (13.98, 14.06) -> (13.98, 6.44)
  line L9 (16.52, 14.06) -> (16.52, 6.44)
  line L10 (19.06, 14.06) -> (19.06, 6.44)
  line L11 (21.6, 14.06) -> (21.6, 6.44)
  line L12 (24.14, 14.06) -> (24.14, 6.44)
  line L13 (26.68, 14.06) -> (26.68, 6.44)
  line L14 (-24.12, 19.14) -> (-24.12, 6.44)
  circle A0 centre (-13.96, -16.42) radius 0.5
  line L15 (-11.42, 19.14) -> (-8.88, 19.14)
  line L16 (-11.42, 14.06) -> (-11.42, 16.6)
  line L17 (1.28, 14.06) -> (1.28, 6.44)
  line L18 (-1.26, 14.06) -> (-1.26, 6.44)
  line L19 (-3.8, 14.06) -> (-3.8, 6.44)
  line L20 (-6.34, 14.06) -> (-6.34, 6.44)
  line L21 (-8.88, 14.06) -> (-8.88, 6.44)
  line L22 (3.82, 14.06) -> (3.82, 11.52)
  line L23 (8.9, -8.8) -> (8.9, -16.42)
  line L24 (11.44, -8.8) -> (11.44, -16.42)
  line L25 (13.98, -8.8) -> (13.98, -16.42)
  line L26 (16.52, -8.8) -> (16.52, -16.42)
  line L27 (19.06, -8.8) -> (19.06, -16.42)
  line L28 (21.6, -8.8) -> (21.6, -16.42)
  line L29 (24.14, -8.8) -> (24.14, -16.42)
  line L30 (26.68, -8.8) -> (26.68, -16.42)
  line L31 (29.22, -8.8) -> (29.22, -16.42)
  line L32 (32.2, 3.91) -> (32.2, -16.41)
  line L33 (-29.2, -18.96) -> (-29.2, -8.8)
  line L34 (-24.12, -18.96) -> (-24.12, -21.5)
  line L35 (6.36, 21.68) -> (6.36, 14.06)
  line L36 (-19.04, -16.42) -> (-21.58, -8.8)
  line L37 (-16.5, -16.42) -> (-19.04, -8.8)
  line L38 (-13.96, -16.42) -> (-16.5, -8.8)
  line L39 (-11.42, -8.8) -> (-11.42, -16.42)
  line L40 (3.82, -8.8) -> (3.82, -16.42)
  line L41 (1.28, -8.8) -> (1.28, -16.42)
  line L42 (-1.26, -8.8) -> (-1.26, -16.42)
  line L43 (-3.8, -8.8) -> (-3.8, -16.42)
  line L44 (-6.34, -16.42) -> (-6.34, -18.96)
  line L45 (-8.88, -16.42) -> (-8.88, -18.96)
  point P0 (29.22, 6.44)
  point P1 (32.2, 3.91)
  point P2 (6.36, 6.44)
  point P3 (3.82, 6.44)
  point P4 (-21.58, 19.14)
  point P5 (-21.58, 6.44)
  point P6 (-19.04, 19.14)
  point P7 (-19.04, 6.44)
  point P8 (-16.5, 19.14)
  point P9 (-16.5, 6.44)
  point P10 (-13.96, 19.14)
  point P11 (-13.96, 6.44)
  point P12 (6.36, 14.06)
  point P13 (1.28, 6.44)
  point P14 (-1.26, 6.44)
  point P15 (-3.8, 6.44)
  point P16 (-6.34, 6.44)
  point P17 (-8.88, 6.44)
  point P18 (8.9, 14.06)
  point P19 (8.9, 6.44)
  point P20 (11.44, 14.06)
  point P21 (11.44, 6.44)
  point P22 (13.98, 14.06)
  point P23 (13.98, 6.44)
  point P24 (16.52, 14.06)
  point P25 (16.52, 6.44)
  point P26 (19.06, 14.06)
  point P27 (19.06, 6.44)
  point P28 (21.6, 14.06)
  point P29 (21.6, 6.44)
  point P30 (24.14, 14.06)
  point P31 (24.14, 6.44)
  point P32 (26.68, 14.06)
  point P33 (26.68, 6.44)
  point P34 (8.9, -8.8)
  point P35 (11.44, -8.8)
  point P36 (13.98, -8.8)
  point P37 (16.52, -8.8)
  point P38 (19.06, -8.8)
  point P39 (21.6, -8.8)
  point P40 (24.14, -8.8)
  point P41 (26.68, -8.8)
  point P42 (29.22, -8.8)
  point P43 (-8.88, 14.06)
  point P44 (-6.34, 14.06)
  point P45 (-3.8, 14.06)
  point P46 (-1.26, 14.06)
  point P47 (1.28, 14.06)
  point P48 (8.9, -16.42)
  point P49 (11.44, -16.42)
  point P50 (13.98, -16.42)
  point P51 (16.52, -16.42)
  point P52 (19.06, -16.42)
  point P53 (21.6, -16.42)
  point P54 (24.14, -16.42)
  point P55 (26.68, -16.42)
  point P56 (29.22, -16.42)
  point P57 (32.2, -16.41)
  point P58 (-19.04, -16.42)
  point P59 (-21.58, -8.8)
  point P60 (-16.5, -16.42)
  point P61 (-19.04, -8.8)
  point P62 (-16.5, -8.8)
  point P63 (-11.42, -8.8)
  point P64 (-11.42, -16.42)
  point P65 (3.82, -8.8)
  point P66 (3.82, -16.42)
  point P67 (1.28, -8.8)
  point P68 (1.28, -16.42)
  point P69 (-1.26, -8.8)
  point P70 (-1.26, -16.42)
  point P71 (-3.8, -8.8)
  point P72 (-3.8, -16.42)
  constraint coincident P0 L0.start
  constraint coincident P1 L0.end
  constraint coincident P4 L1.start
  constraint coincident P5 L1.end
  constraint coincident P6 L2.start
  constraint coincident P7 L2.end
  constraint coincident P8 L3.start
  constraint coincident P9 L3.end
  constraint coincident P10 L4.start
  constraint coincident P11 L4.end
  constraint coincident P12 L5.start
  constraint coincident P2 L5.end
  constraint coincident P18 L6.start
  constraint coincident P19 L6.end
  constraint coincident P20 L7.start
  constraint coincident P21 L7.end
  constraint coincident P22 L8.start
  constraint coincident P23 L8.end
  constraint coincident P24 L9.start
  constraint coincident P25 L9.end
  constraint coincident P26 L10.start
  constraint coincident P27 L10.end
  constraint coincident P28 L11.start
  constraint coincident P29 L11.end
  constraint coincident P30 L12.start
  constraint coincident P31 L12.end
  constraint coincident P32 L13.start
  constraint coincident P33 L13.end
  constraint coincident P47 L17.start
  constraint coincident P13 L17.end
  constraint coincident P46 L18.start
  constraint coincident P14 L18.end
  constraint coincident P45 L19.start
  constraint coincident P15 L19.end
  constraint coincident P44 L20.start
  constraint coincident P16 L20.end
  constraint coincident P43 L21.start
  constraint coincident P17 L21.end
  constraint coincident P34 L23.start
  constraint coincident P48 L23.end
  constraint coincident P35 L24.start
  constraint coincident P49 L24.end
  constraint coincident P36 L25.start
  constraint coincident P50 L25.end
  constraint coincident P37 L26.start
  constraint coincident P51 L26.end
  constraint coincident P38 L27.start
  constraint coincident P52 L27.end
  constraint coincident P39 L28.start
  constraint coincident P53 L28.end
  constraint coincident P40 L29.start
  constraint coincident P54 L29.end
  constraint coincident P41 L30.start
  constraint coincident P55 L30.end
  constraint coincident P42 L31.start
  constraint coincident P56 L31.end
  constraint coincident P57 L32.end
  constraint coincident P58 L36.start
  constraint coincident P59 L36.end
  constraint coincident P60 L37.start
  constraint coincident P61 L37.end
  constraint coincident A0.centre L38.start
  constraint coincident P62 L38.end
  constraint coincident P63 L39.start
  constraint coincident P64 L39.end
  constraint coincident P65 L40.start
  constraint coincident P66 L40.end
  constraint coincident P67 L41.start
  constraint coincident P68 L41.end
  constraint coincident P69 L42.start
  constraint coincident P70 L42.end
  constraint coincident P71 L43.start
  constraint coincident P72 L43.end
sketch "top wires" plane through (0, 0, 0) normal (0, 0, 1) x (1, 0, 0)
  line L0 (6.36, 16.6) -> (6.36, 14.06)
  line L1 (-8.88, 19.14) -> (-11.42, 19.14)
  line L2 (-24.12, 11.52) -> (3.82, 11.52)
  line L3 (3.82, 14.06) -> (3.82, 11.52)
  line L4 (-24.12, 19.14) -> (-24.12, 11.52)
  line L5 (-24.12, 11.52) -> (-24.12, 6.44)
  line L6 (-11.42, 16.6) -> (-11.42, 14.06)
  line L7 (-29.2, 8.98) -> (-29.2, 6.44)
  line L8 (-29.2, 11.52) -> (-29.2, 8.98)
  arc A0 (-11.42, 16.6) -> (-29.2, 11.52) centre (-11.1633, -17.9536) ccw
  arc A1 (-29.2, 8.98) -> (-32.2, 6.45) centre (-29.4125, 6.1883) ccw
  line L9 (-32.2, 6.45) -> (-32.2, -18.95)
  arc A2 (-32.2, -18.95) -> (-29.2, -21.5) centre (-29.6162, -18.95) ccw
  line L10 (-29.2, -21.5) -> (-24.12, -21.5)
  line L11 (-24.12, -18.96) -> (-24.12, -21.5)
  line L12 (-24.12, -21.5) -> (-24.12, -18.96)
  line L13 (-24.12, -18.96) -> (-24.12, -21.5)
  arc A3 (-8.88, 19.14) -> (6.36, 16.6) centre (1.28, 33.11) ccw
  line L14 (6.36, 16.6) -> (6.36, 21.68)
  spline S0 degree 5 poles (-26.66, -16.42) (-26.5297, -16.4351) (-26.2708, -16.4682) (-25.8873, -16.5263) (-25.3857, -16.621) (-24.7755, -16.7684) (-24.1828, -16.9445) (-23.6088, -17.1478) (-23.0543, -17.3747) (-22.5205, -17.618) (-22.0078, -17.8677) (-21.5171, -18.112) (-21.0485, -18.3392) (-20.6025, -18.539) (-20.1787, -18.7041) (-19.7766, -18.8313) (-19.4717, -18.902) (-19.2523, -18.9377) (-19.1101, -18.9538) (-19.04, -18.96) knots 0 0 0 0 0 0 0.066667 0.133333 0.2 0.266667 0.333333 0.4 0.466667 0.533333 0.6 0.666667 0.733333 0.8 0.866667 0.933333 1 1 1 1 1 1
  circle A4 centre (-19.04, -18.96) radius 0.5
  line L15 (-26.66, -16.42) -> (-29.2, -16.42)
  line L16 (-29.2, -16.42) -> (-29.2, -8.8)
  line L17 (-29.2, -8.8) -> (-29.2, -16.42)
  line L18 (-19.04, -18.96) -> (-8.88, -18.96)
  line L19 (-8.88, -18.96) -> (-8.88, -16.42)
  arc A5 (-6.34, -18.96) -> (6.36, -18.96) centre (0.01, -7.7481) ccw
  arc A6 (6.36, -18.96) -> (6.36, -18) centre (6.0881, -18.48) ccw
  line L20 (6.36, -18) -> (6.36, -8.8)
  line L21 (6.36, -8.8) -> (6.36, -11.34)
  line L22 (-6.34, -18.96) -> (-6.34, -16.42)
  point P0 (-8.88, 19.14)
  point P1 (6.36, 16.6)
  point P2 (6.36, 14.06)
  point P3 (-11.42, 19.14)
  point P4 (-24.12, 11.52)
  point P5 (3.82, 11.52)
  point P6 (3.82, 14.06)
  point P7 (-24.12, 19.14)
  point P8 (-24.12, 6.44)
  point P9 (-29.2, 8.98)
  point P10 (-11.42, 16.6)
  point P11 (-11.42, 14.06)
  point P12 (-29.2, 6.44)
  point P13 (-29.2, 11.52)
  point P14 (-24.12, -18.96)
  point P15 (-3.8, 16.6)
  point P16 (6.36, 21.68)
  point P17 (-23.2903, -17.2817)
  point P18 (-20.739, -18.4745)
  point P19 (-26.66, -16.42)
  point P20 (-19.04, -18.96)
  point P21 (-29.2, -16.42)
  point P22 (-29.2, -8.8)
  point P23 (-8.88, -18.96)
  point P24 (-8.88, -16.42)
  point P25 (-6.34, -18.96)
  point P26 (6.36, -18.96)
  point P27 (6.36, -8.8)
  point P28 (6.36, -11.34)
  point P29 (-6.34, -16.42)
  constraint coincident L0.start A3.end
  constraint coincident P2 L0.end
  constraint coincident P0 L1.start
  constraint coincident P3 L1.end
  constraint coincident P4 L2.start
  constraint coincident P5 L2.end
  constraint coincident P6 L3.start
  constraint coincident P7 L4.start
  constraint coincident P8 L5.end
  constraint coincident P10 L6.start
  constraint coincident P9 L7.start
  constraint coincident P11 L6.end
  constraint coincident P12 L7.end
  constraint coincident P13 L8.start
  constraint tangent L9 A2
  constraint coincident P14 L11.start
  constraint perpendicular L10 L11
  constraint coincident A3 P15
  constraint coincident P1 L0.start
  constraint coincident P16 L14.end
  constraint coincident P19 S0.start
  constraint coincident P20 S0.end
  constraint coincident P21 L15.end
  constraint perpendicular L9 L15
  constraint coincident P22 L16.end
  constraint coincident P23 L18.end
  constraint coincident P24 L19.end
  constraint coincident P26 A5.end
  constraint coincident P25 A5.start
  constraint tangent A5 A6
  constraint coincident P27 L20.end
  constraint coincident P28 L21.end
  constraint coincident P29 L22.end
sketch "bottom wires" plane through (0, 0, 0) normal (0, 0, 1) x (1, 0, 0)
  arc A0 (-13.96, -8.8) -> (-28, -8.8) centre (-20.98, -11.0359) ccw
  line L0 (-28, -8.8) -> (-26.66, -18.96)
  arc A1 (-8.88, -8.8) -> (0, 5) centre (-19.3481, 7.693) ccw
  arc A2 (-6.34, -8.8) -> (2.5296, 5.0052) centre (-14.7149, 6.3326) ccw
  line L1 (0, 5) -> (0, 19)
  line L2 (2.5296, 5.0052) -> (2.5296, 19)
  arc A3 (1.28, 21.68) -> (0, 19) centre (3.0691, 19.1798) ccw
  arc A4 (3.82, 21.68) -> (2.5296, 19) centre (5.9578, 19) ccw
  point P0 (3.82, 6.44)
  point P1 (-29.2, 6.44)
  point P2 (-24.12, 6.44)
  point P3 (-13.96, -8.8)
  point P4 (-26.66, -18.96)
  point P5 (-8.88, -8.8)
  point P6 (-6.34, -8.8)
  point P7 (1.28, 21.68)
  point P8 (0.407, 20.7177)
  point P9 (3.82, 21.68)
  constraint coincident P3 A0.start
  constraint coincident P4 L0.end
  constraint coincident P5 A1.start
  constraint coincident P6 A2.start
  constraint vertical L2
  constraint coincident A3 P8
  constraint coincident P7 A3.start
  constraint tangent L2 A4
  constraint coincident P9 A4.start
sketch "additions" plane through (0, 0, 0) normal (0, 0, 1) x (1, 0, 0)
  line L0 (3.82, 6.44) -> (3.82, 3.9)
  line L1 (3.82, 3.9) -> (8.9, 3.9)
  line L2 (8.9, 3.9) -> (8.9, 6.44)
  line L3 (-11.42, 6.44) -> (-11.42, 1.36)
  line L4 (-11.42, 1.36) -> (11.44, 1.36)
  line L5 (11.44, 1.36) -> (11.44, 6.44)
  point P0 (3.82, 6.44)
  point P1 (3.82, 3.9)
  point P2 (8.9, 3.9)
  point P3 (8.9, 6.44)
  point P4 (-11.42, 6.44)
  point P5 (-11.42, 1.36)
  point P6 (11.44, 1.36)
  point P7 (11.44, 6.44)
  constraint coincident P0 L0.start
  constraint coincident P1 L0.end
  constraint coincident P2 L1.end
  constraint coincident P3 L2.end
  constraint coincident P4 L3.start
  constraint coincident P5 L3.end
  constraint coincident P6 L4.end
  constraint coincident P7 L5.end
